Autodesk Fusion 360 part; units mm, degrees
(part 16 of 20)
  spline S45 degree 3 poles (25.501, -787.6508) (25.5046, -787.8666) (25.5109, -788.2453) (25.6995, -788.5712) (25.7807, -788.7115) knots 0 0 0 0 0.063398 0.111295 0.111295 0.111295 0.111295
  spline S46 degree 3 poles (25.7807, -788.7115) (25.8819, -788.808) (26.0864, -789.0031) (26.3682, -789.0291) (26.5106, -789.0423) knots 0 0 0 0 0.040675 0.082263 0.082263 0.082263 0.082263
  spline S47 degree 3 poles (26.5106, -789.0423) (26.625, -789.0341) (26.8478, -789.018) (27.0271, -788.8852) (27.1143, -788.8205) knots 0 0 0 0 0.033628 0.065508 0.065508 0.065508 0.065508
  spline S48 degree 3 poles (27.1143, -788.8205) (27.1883, -788.7306) (27.3518, -788.5319) (27.3967, -788.2775) (27.4212, -788.1384) knots 0 0 0 0 0.034396 0.07593 0.07593 0.07593 0.07593
  spline S49 degree 3 poles (21.7321, -737.034) (21.7357, -736.7657) (21.7422, -736.2825) (21.8615, -735.8147) (21.9145, -735.6066) knots 0 0 0 0 0.080152 0.144341 0.144341 0.144341 0.144341
  spline S50 degree 3 poles (21.9145, -735.6066) (21.9791, -735.4398) (22.1017, -735.1233) (22.3428, -734.8853) (22.4568, -734.7727) knots 0 0 0 0 0.052977 0.10048 0.10048 0.10048 0.10048
  spline S51 degree 3 poles (22.4568, -734.7727) (22.5882, -734.6872) (22.863, -734.5083) (23.1911, -734.4893) (23.3623, -734.4794) knots 0 0 0 0 0.046203 0.096661 0.096661 0.096661 0.096661
  spline S52 degree 3 poles (23.3623, -734.4794) (23.4901, -734.485) (23.7356, -734.4957) (23.9605, -734.5941) (24.0683, -734.6414) knots 0 0 0 0 0.037989 0.072993 0.072993 0.072993 0.072993
  spline S53 degree 3 poles (24.0683, -734.6414) (24.1655, -734.7021) (24.3629, -734.8252) (24.5001, -735.0132) (24.5697, -735.1086) knots 0 0 0 0 0.034048 0.069103 0.069103 0.069103 0.069103
  spline S54 degree 3 poles (24.5697, -735.1086) (24.633, -735.2196) (24.767, -735.4545) (24.841, -735.7148) (24.8801, -735.8521) knots 0 0 0 0 0.038176 0.080832 0.080832 0.080832 0.080832
  spline S55 degree 3 poles (24.8801, -735.8521) (24.9128, -736.0232) (24.9874, -736.4133) (24.9907, -736.8107) (24.9926, -737.0339) knots 0 0 0 0 0.052146 0.118926 0.118926 0.118926 0.118926
  spline S56 degree 3 poles (24.9926, -737.0339) (24.989, -737.3005) (24.9824, -737.7813) (24.8645, -738.247) (24.8119, -738.4544) knots 0 0 0 0 0.079639 0.143634 0.143634 0.143634 0.143634
  spline S57 degree 3 poles (24.8119, -738.4544) (24.7477, -738.6214) (24.6259, -738.9384) (24.3852, -739.1771) (24.2713, -739.2901) knots 0 0 0 0 0.052961 0.100531 0.100531 0.100531 0.100531
  spline S58 degree 3 poles (24.2713, -739.2901) (24.1397, -739.3761) (23.864, -739.5562) (23.5346, -739.5752) (23.3624, -739.5851) knots 0 0 0 0 0.046339 0.097057 0.097057 0.097057 0.097057
  spline S59 degree 3 poles (23.3624, -739.5851) (23.1362, -739.5658) (22.6949, -739.5281) (22.3801, -739.2179) (22.2267, -739.0667) knots 0 0 0 0 0.065835 0.128409 0.128409 0.128409 0.128409
  spline S60 degree 3 poles (22.2267, -739.0667) (22.0832, -738.7986) (21.7456, -738.1676) (21.737, -737.4479) (21.7321, -737.034) knots 0 0 0 0 0.090022 0.211899 0.211899 0.211899 0.211899
  line L356 (28.1509, -738.173) -> (28.7546, -738.2514)
  spline S61 degree 3 poles (28.7546, -738.2514) (28.7119, -738.4453) (28.6302, -738.8171) (28.3717, -739.0954) (28.2481, -739.2286) knots 0 0 0 0 0.058356 0.111856 0.111856 0.111856 0.111856
  spline S62 degree 3 poles (28.2481, -739.2286) (28.1021, -739.3315) (27.802, -739.543) (27.4353, -739.5685) (27.2471, -739.5816) knots 0 0 0 0 0.052559 0.107965 0.107965 0.107965 0.107965
  spline S63 degree 3 poles (27.2471, -739.5816) (27.0141, -739.5641) (26.5625, -739.5302) (26.2182, -739.2373) (26.0517, -739.0956) knots 0 0 0 0 0.068154 0.132052 0.132052 0.132052 0.132052
  spline S64 degree 3 poles (26.0517, -739.0956) (25.9201, -738.9049) (25.6323, -738.4875) (25.6112, -737.9787) (25.5997, -737.7024) knots 0 0 0 0 0.068157 0.149141 0.149141 0.149141 0.149141
  spline S65 degree 3 poles (25.5997, -737.7024) (25.6061, -737.5171) (25.6181, -737.1646) (25.7375, -736.8331) (25.7941, -736.6758) knots 0 0 0 0 0.055211 0.105055 0.105055 0.105055 0.105055
  spline S66 degree 3 poles (25.7941, -736.6758) (25.8663, -736.5389) (26.0085, -736.2693) (26.2614, -736.0994) (26.3859, -736.0158) knots 0 0 0 0 0.04564 0.089884 0.089884 0.089884 0.089884
  spline S67 degree 3 poles (26.3859, -736.0158) (26.5218, -735.9516) (26.7957, -735.8223) (27.0981, -735.8047) (27.2505, -735.7958) knots 0 0 0 0 0.044643 0.089956 0.089956 0.089956 0.089956
  spline S68 degree 3 poles (27.2505, -735.7958) (27.4342, -735.8052) (27.7821, -735.8229) (28.0767, -736.0072) (28.2157, -736.0942) knots 0 0 0 0 0.054149 0.102527 0.102527 0.102527 0.102527
  spline S69 degree 3 poles (28.2157, -736.0942) (28.3301, -736.2077) (28.5692, -736.4447) (28.6529, -736.7715) (28.6966, -736.9417) knots 0 0 0 0 0.047449 0.099081 0.099081 0.099081 0.099081
  line L357 (28.6966, -736.9417) -> (28.0997, -737.0338)
  spline S70 degree 3 poles (28.0997, -737.0338) (28.0689, -736.9224) (28.0114, -736.715) (27.8654, -736.5576) (27.7979, -736.4847) knots 0 0 0 0 0.034086 0.063475 0.063475 0.063475 0.063475
  spline S71 degree 3 poles (27.7979, -736.4847) (27.7209, -736.431) (27.5636, -736.3213) (27.3721, -736.3076) (27.2743, -736.3006) knots 0 0 0 0 0.027619 0.056426 0.056426 0.056426 0.056426
  spline S72 degree 3 poles (27.2743, -736.3006) (27.1277, -736.3136) (26.8385, -736.3393) (26.6256, -736.5361) (26.5206, -736.6331) knots 0 0 0 0 0.04285 0.084486 0.084486 0.084486 0.084486
  spline S73 degree 3 poles (26.5206, -736.6331) (26.4364, -736.7727) (26.2425, -737.0942) (26.235, -737.4717) (26.2307, -737.6853) knots 0 0 0 0 0.048123 0.11083 0.11083 0.11083 0.11083
  spline S74 degree 3 poles (26.2307, -737.6853) (26.2343, -737.9011) (26.2406, -738.2798) (26.4292, -738.6057) (26.5104, -738.746) knots 0 0 0 0 0.063398 0.111295 0.111295 0.111295 0.111295
  spline S75 degree 3 poles (26.5104, -738.746) (26.6116, -738.8425) (26.8161, -739.0376) (27.0979, -739.0637) (27.2403, -739.0768) knots 0 0 0 0 0.040675 0.082263 0.082263 0.082263 0.082263
  spline S76 degree 3 poles (27.2403, -739.0768) (27.3547, -739.0686) (27.5775, -739.0526) (27.7568, -738.9198) (27.844, -738.8551) knots 0 0 0 0 0.033628 0.065508 0.065508 0.065508 0.065508
  spline S77 degree 3 poles (27.844, -738.8551) (27.918, -738.7651) (28.0815, -738.5665) (28.1264, -738.3121) (28.1509, -738.173) knots 0 0 0 0 0.034396 0.07593 0.07593 0.07593 0.07593
  line L358 (21.7306, -688.1902) -> (22.3752, -688.1357)
  spline S78 degree 3 poles (22.3752, -688.1357) (22.4029, -688.2789) (22.4541, -688.5438) (22.6279, -688.7491) (22.7077, -688.8434) knots 0 0 0 0 0.042908 0.079365 0.079365 0.079365 0.079365
  spline S79 degree 3 poles (22.7077, -688.8434) (22.7999, -688.9125) (22.9865, -689.0525) (23.2192, -689.071) (23.337, -689.0804) knots 0 0 0 0 0.033826 0.068485 0.068485 0.068485 0.068485
  spline S80 degree 3 poles (23.337, -689.0804) (23.4794, -689.0661) (23.7662, -689.0373) (23.9798, -688.8436) (24.0873, -688.7462) knots 0 0 0 0 0.041772 0.0841 0.0841 0.0841 0.0841
  spline S81 degree 3 poles (24.0873, -688.7462) (24.1768, -688.6211) (24.366, -688.3566) (24.3845, -688.031) (24.3943, -687.8594) knots 0 0 0 0 0.045186 0.095569 0.095569 0.095569 0.095569
  spline S82 degree 3 poles (24.3943, -687.8594) (24.3852, -687.697) (24.3681, -687.3907) (24.1852, -687.1457) (24.0992, -687.0306) knots 0 0 0 0 0.047557 0.089725 0.089725 0.089725 0.089725
  spline S83 degree 3 poles (24.0992, -687.0306) (23.9907, -686.9421) (23.7662, -686.7589) (23.4765, -686.7379) (23.3267, -686.7271) knots 0 0 0 0 0.040971 0.08482 0.08482 0.08482 0.08482
  spline S84 degree 3 poles (23.3267, -686.7271) (23.2311, -686.7322) (23.0437, -686.7423) (22.8742, -686.8225) (22.7912, -686.8618) knots 0 0 0 0 0.028423 0.055689 0.055689 0.055689 0.055689
  spline S85 degree 3 poles (22.7912, -686.8618) (22.7164, -686.9093) (22.5695, -687.0026) (22.4666, -687.1427) (22.4161, -687.2114) knots 0 0 0 0 0.026342 0.051681 0.051681 0.051681 0.051681
  line L359 (22.4161, -687.2114) -> (21.8397, -687.1364)
  line L360 (21.8397, -687.1364) -> (22.324, -684.5681)
  line L361 (22.324, -684.5681) -> (24.8103, -684.5681)
  line L362 (24.8103, -684.5681) -> (24.8103, -685.1547)
  line L363 (24.8103, -685.1547) -> (22.8151, -685.1548)
  line L364 (22.8151, -685.1548) -> (22.5457, -686.4986)
  spline S86 degree 3 poles (22.5457, -686.4986) (22.6952, -686.4071) (22.986, -686.229) (23.3254, -686.1992) (23.4904, -686.1848) knots 0 0 0 0 0.051785 0.100763 0.100763 0.100763 0.100763
  spline S87 degree 3 poles (23.4904, -686.1848) (23.6997, -686.2031) (24.1153, -686.2396) (24.4361, -686.5061) (24.5955, -686.6384) knots 0 0 0 0 0.061424 0.122014 0.122014 0.122014 0.122014
  spline S88 degree 3 poles (24.5955, -686.6384) (24.7267, -686.8038) (24.9976, -687.1451) (25.0293, -687.5805) (25.0457, -687.8048) knots 0 0 0 0 0.061868 0.127641 0.127641 0.127641 0.127641
  spline S89 degree 3 poles (25.0457, -687.8048) (25.0305, -688.0218) (25.0006, -688.4476) (24.7654, -688.8035) (24.6501, -688.9781) knots 0 0 0 0 0.064036 0.125703 0.125703 0.125703 0.125703
  spline S90 degree 3 poles (24.6501, -688.9781) (24.4723, -689.1551) (24.1093, -689.5168) (23.598, -689.5621) (23.337, -689.5852) knots 0 0 0 0 0.072854 0.148822 0.148822 0.148822 0.148822
  spline S91 degree 3 poles (23.337, -689.5852) (23.1238, -689.5724) (22.7162, -689.5481) (22.3825, -689.3145) (22.2234, -689.2032) knots 0 0 0 0 0.062678 0.119794 0.119794 0.119794 0.119794
  spline S92 degree 3 poles (22.2234, -689.2032) (22.0948, -689.0628) (21.8305, -688.7745) (21.7644, -688.3884) (21.7306, -688.1902) knots 0 0 0 0 0.055877 0.114795 0.114795 0.114795 0.114795
  line L365 (28.1494, -688.1731) -> (28.7531, -688.2516)
  spline S93 degree 3 poles (28.7531, -688.2516) (28.7104, -688.4455) (28.6286, -688.8172) (28.3702, -689.0956) (28.2466, -689.2287) knots 0 0 0 0 0.058356 0.111856 0.111856 0.111856 0.111856
  spline S94 degree 3 poles (28.2466, -689.2287) (28.1005, -689.3317) (27.8004, -689.5431) (27.4337, -689.5686) (27.2456, -689.5817) knots 0 0 0 0 0.052559 0.107965 0.107965 0.107965 0.107965
  spline S95 degree 3 poles (27.2456, -689.5817) (27.0125, -689.5642) (26.5609, -689.5303) (26.2167, -689.2374) (26.0501, -689.0957) knots 0 0 0 0 0.068154 0.132052 0.132052 0.132052 0.132052
  spline S96 degree 3 poles (26.0501, -689.0957) (25.9186, -688.905) (25.6307, -688.4876) (25.6097, -687.9788) (25.5982, -687.7025) knots 0 0 0 0 0.068157 0.149141 0.149141 0.149141 0.149141
  spline S97 degree 3 poles (25.5982, -687.7025) (25.6045, -687.5172) (25.6165, -687.1647) (25.7359, -686.8332) (25.7926, -686.6759) knots 0 0 0 0 0.055211 0.105055 0.105055 0.105055 0.105055
  spline S98 degree 3 poles (25.7926, -686.6759) (25.8648, -686.539) (26.007, -686.2694) (26.2599, -686.0995) (26.3843, -686.0159) knots 0 0 0 0 0.04564 0.089884 0.089884 0.089884 0.089884
  spline S99 degree 3 poles (26.3843, -686.0159) (26.5203, -685.9517) (26.7942, -685.8225) (27.0966, -685.8048) (27.2489, -685.7959) knots 0 0 0 0 0.044643 0.089955 0.089955 0.089955 0.089955
  spline S100 degree 3 poles (27.2489, -685.7959) (27.4327, -685.8053) (27.7805, -685.8231) (28.0751, -686.0074) (28.2142, -686.0943) knots 0 0 0 0 0.054149 0.102527 0.102527 0.102527 0.102527
  spline S101 degree 3 poles (28.2142, -686.0943) (28.3286, -686.2078) (28.5677, -686.4449) (28.6514, -686.7716) (28.6951, -686.9419) knots 0 0 0 0 0.047449 0.099081 0.099081 0.099081 0.099081
  line L366 (28.6951, -686.9419) -> (28.0982, -687.034)
  spline S102 degree 3 poles (28.0982, -687.034) (28.0673, -686.9226) (28.0099, -686.7151) (27.8639, -686.5577) (27.7964, -686.4849) knots 0 0 0 0 0.034086 0.063475 0.063475 0.063475 0.063475
  spline S103 degree 3 poles (27.7964, -686.4849) (27.7194, -686.4311) (27.5621, -686.3214) (27.3706, -686.3077) (27.2728, -686.3007) knots 0 0 0 0 0.027619 0.056426 0.056426 0.056426 0.056426
  spline S104 degree 3 poles (27.2728, -686.3007) (27.1262, -686.3137) (26.837, -686.3394) (26.624, -686.5362) (26.5191, -686.6332) knots 0 0 0 0 0.04285 0.084486 0.084486 0.084486 0.084486
  spline S105 degree 3 poles (26.5191, -686.6332) (26.4349, -686.7728) (26.241, -687.0943) (26.2335, -687.4718) (26.2292, -687.6854) knots 0 0 0 0 0.048123 0.11083 0.11083 0.11083 0.11083
  spline S106 degree 3 poles (26.2292, -687.6854) (26.2328, -687.9012) (26.2391, -688.2799) (26.4277, -688.6059) (26.5089, -688.7461) knots 0 0 0 0 0.063398 0.111295 0.111295 0.111295 0.111295
  spline S107 degree 3 poles (26.5089, -688.7461) (26.61, -688.8426) (26.8146, -689.0378) (27.0963, -689.0638) (27.2387, -689.0769) knots 0 0 0 0 0.040675 0.082263 0.082263 0.082263 0.082263
  spline S108 degree 3 poles (27.2387, -689.0769) (27.3531, -689.0687) (27.576, -689.0527) (27.7552, -688.9199) (27.8424, -688.8553) knots 0 0 0 0 0.033628 0.065508 0.065508 0.065508 0.065508
  spline S109 degree 3 poles (27.8424, -688.8553) (27.9165, -688.7653) (28.0799, -688.5666) (28.1248, -688.3123) (28.1494, -688.1731) knots 0 0 0 0 0.034396 0.07593 0.07593 0.07593 0.07593
  spline S110 degree 3 poles (22.0101, -637.034) (22.0137, -636.7656) (22.0202, -636.2824) (22.1394, -635.8146) (22.1925, -635.6066) knots 0 0 0 0 0.080152 0.144341 0.144341 0.144341 0.144341
  spline S111 degree 3 poles (22.1925, -635.6066) (22.2571, -635.4397) (22.3796, -635.1233) (22.6208, -634.8852) (22.7348, -634.7727) knots 0 0 0 0 0.052977 0.10048 0.10048 0.10048 0.10048
  spline S112 degree 3 poles (22.7348, -634.7727) (22.8661, -634.6872) (23.141, -634.5083) (23.469, -634.4893) (23.6403, -634.4794) knots 0 0 0 0 0.046203 0.096661 0.096661 0.096661 0.096661
  spline S113 degree 3 poles (23.6403, -634.4794) (23.7681, -634.4849) (24.0136, -634.4956) (24.2384, -634.5941) (24.3463, -634.6413) knots 0 0 0 0 0.037989 0.072993 0.072993 0.072993 0.072993
  spline S114 degree 3 poles (24.3463, -634.6413) (24.4435, -634.702) (24.6409, -634.8252) (24.7781, -635.0132) (24.8477, -635.1086) knots 0 0 0 0 0.034048 0.069103 0.069103 0.069103 0.069103
  spline S115 degree 3 poles (24.8477, -635.1086) (24.911, -635.2195) (25.045, -635.4544) (25.119, -635.7147) (25.1581, -635.8521) knots 0 0 0 0 0.038176 0.080832 0.080832 0.080832 0.080832
  spline S116 degree 3 poles (25.1581, -635.8521) (25.1908, -636.0231) (25.2653, -636.4133) (25.2687, -636.8107) (25.2706, -637.0339) knots 0 0 0 0 0.052146 0.118926 0.118926 0.118926 0.118926
  spline S117 degree 3 poles (25.2706, -637.0339) (25.267, -637.3005) (25.2604, -637.7813) (25.1425, -638.2469) (25.0899, -638.4544) knots 0 0 0 0 0.079639 0.143634 0.143634 0.143634 0.143634
  spline S118 degree 3 poles (25.0899, -638.4544) (25.0257, -638.6214) (24.9039, -638.9383) (24.6632, -639.1771) (24.5493, -639.29) knots 0 0 0 0 0.052961 0.100531 0.100531 0.100531 0.100531
  spline S119 degree 3 poles (24.5493, -639.29) (24.4177, -639.376) (24.142, -639.5562) (23.8126, -639.5752) (23.6404, -639.5851) knots 0 0 0 0 0.046339 0.097057 0.097057 0.097057 0.097057
  spline S120 degree 3 poles (23.6404, -639.5851) (23.4142, -639.5658) (22.9729, -639.5281) (22.6581, -639.2179) (22.5047, -639.0667) knots 0 0 0 0 0.065835 0.128409 0.128409 0.128409 0.128409
  spline S121 degree 3 poles (22.5047, -639.0667) (22.3612, -638.7986) (22.0236, -638.1676) (22.015, -637.4479) (22.0101, -637.034) knots 0 0 0 0 0.090022 0.211899 0.211899 0.211899 0.211899
  line L367 (28.4289, -638.1729) -> (29.0326, -638.2514)
  spline S122 degree 3 poles (29.0326, -638.2514) (28.9899, -638.4453) (28.9082, -638.817) (28.6498, -639.0954) (28.5262, -639.2285) knots 0 0 0 0 0.058356 0.111856 0.111856 0.111856 0.111856
  spline S123 degree 3 poles (28.5262, -639.2285) (28.3801, -639.3315) (28.08, -639.5429) (27.7133, -639.5685) (27.5251, -639.5816) knots 0 0 0 0 0.052559 0.107965 0.107965 0.107965 0.107965
  spline S124 degree 3 poles (27.5251, -639.5816) (27.2921, -639.5641) (26.8405, -639.5301) (26.4963, -639.2373) (26.3297, -639.0956) knots 0 0 0 0 0.068154 0.132052 0.132052 0.132052 0.132052
  spline S125 degree 3 poles (26.3297, -639.0956) (26.1981, -638.9048) (25.9103, -638.4875) (25.8892, -637.9786) (25.8777, -637.7023) knots 0 0 0 0 0.068157 0.149141 0.149141 0.149141 0.149141
  spline S126 degree 3 poles (25.8777, -637.7023) (25.8841, -637.5171) (25.8961, -637.1646) (26.0155, -636.833) (26.0721, -636.6757) knots 0 0 0 0 0.055211 0.105055 0.105055 0.105055 0.105055
  spline S127 degree 3 poles (26.0721, -636.6757) (26.1443, -636.5388) (26.2865, -636.2692) (26.5394, -636.0994) (26.6639, -636.0158) knots 0 0 0 0 0.04564 0.089884 0.089884 0.089884 0.089884
  spline S128 degree 3 poles (26.6639, -636.0158) (26.7998, -635.9516) (27.0737, -635.8223) (27.3761, -635.8046) (27.5284, -635.7958) knots 0 0 0 0 0.044643 0.089955 0.089955 0.089955 0.089955
  spline S129 degree 3 poles (27.5284, -635.7958) (27.7122, -635.8051) (28.0601, -635.8229) (28.3547, -636.0072) (28.4937, -636.0942) knots 0 0 0 0 0.054149 0.102527 0.102527 0.102527 0.102527
  spline S130 degree 3 poles (28.4937, -636.0942) (28.6081, -636.2077) (28.8472, -636.4447) (28.9309, -636.7714) (28.9746, -636.9417) knots 0 0 0 0 0.047449 0.099081 0.099081 0.099081 0.099081
  line L368 (28.9746, -636.9417) -> (28.3777, -637.0338)
  spline S131 degree 3 poles (28.3777, -637.0338) (28.3469, -636.9224) (28.2894, -636.715) (28.1434, -636.5576) (28.0759, -636.4847) knots 0 0 0 0 0.034086 0.063475 0.063475 0.063475 0.063475
  spline S132 degree 3 poles (28.0759, -636.4847) (27.9989, -636.431) (27.8416, -636.3213) (27.6501, -636.3075) (27.5523, -636.3005) knots 0 0 0 0 0.027619 0.056426 0.056426 0.056426 0.056426
  spline S133 degree 3 poles (27.5523, -636.3005) (27.4057, -636.3136) (27.1165, -636.3393) (26.9036, -636.5361) (26.7986, -636.6331) knots 0 0 0 0 0.04285 0.084486 0.084486 0.084486 0.084486
  spline S134 degree 3 poles (26.7986, -636.6331) (26.7144, -636.7727) (26.5205, -637.0941) (26.513, -637.4717) (26.5087, -637.6853) knots 0 0 0 0 0.048123 0.11083 0.11083 0.11083 0.11083
  spline S135 degree 3 poles (26.5087, -637.6853) (26.5123, -637.901) (26.5186, -638.2798) (26.7072, -638.6057) (26.7884, -638.746) knots 0 0 0 0 0.063398 0.111295 0.111295 0.111295 0.111295
  spline S136 degree 3 poles (26.7884, -638.746) (26.8896, -638.8425) (27.0941, -639.0376) (27.3759, -639.0636) (27.5183, -639.0768) knots 0 0 0 0 0.040675 0.082263 0.082263 0.082263 0.082263
  spline S137 degree 3 poles (27.5183, -639.0768) (27.6327, -639.0686) (27.8555, -639.0526) (28.0348, -638.9197) (28.122, -638.8551) knots 0 0 0 0 0.033628 0.065508 0.065508 0.065508 0.065508
  spline S138 degree 3 poles (28.122, -638.8551) (28.196, -638.7651) (28.3595, -638.5665) (28.4044, -638.3121) (28.4289, -638.1729) knots 0 0 0 0 0.034396 0.07593 0.07593 0.07593 0.07593
  line L369 (22.0076, -588.1903) -> (22.6523, -588.1357)
  spline S139 degree 3 poles (22.6523, -588.1357) (22.68, -588.2789) (22.7312, -588.5439) (22.905, -588.7491) (22.9848, -588.8434) knots 0 0 0 0 0.042908 0.079365 0.079365 0.079365 0.079365
  spline S140 degree 3 poles (22.9848, -588.8434) (23.077, -588.9125) (23.2636, -589.0525) (23.4963, -589.0711) (23.6141, -589.0804) knots 0 0 0 0 0.033826 0.068485 0.068485 0.068485 0.068485
  spline S141 degree 3 poles (23.6141, -589.0804) (23.7565, -589.0662) (24.0433, -589.0374) (24.2569, -588.8437) (24.3644, -588.7462) knots 0 0 0 0 0.041772 0.0841 0.0841 0.0841 0.0841
  spline S142 degree 3 poles (24.3644, -588.7462) (24.4539, -588.6211) (24.6431, -588.3567) (24.6616, -588.0311) (24.6714, -587.8594) knots 0 0 0 0 0.045186 0.095569 0.095569 0.095569 0.095569
  spline S143 degree 3 poles (24.6714, -587.8594) (24.6623, -587.6971) (24.6452, -587.3908) (24.4623, -587.1458) (24.3763, -587.0306) knots 0 0 0 0 0.047557 0.089725 0.089725 0.089725 0.089725
  spline S144 degree 3 poles (24.3763, -587.0306) (24.2678, -586.9421) (24.0433, -586.7589) (23.7536, -586.7379) (23.6038, -586.7271) knots 0 0 0 0 0.040971 0.08482 0.08482 0.08482 0.08482
  spline S145 degree 3 poles (23.6038, -586.7271) (23.5082, -586.7322) (23.3208, -586.7423) (23.1513, -586.8225) (23.0683, -586.8618) knots 0 0 0 0 0.028423 0.055689 0.055689 0.055689 0.055689
  spline S146 degree 3 poles (23.0683, -586.8618) (22.9935, -586.9094) (22.8466, -587.0026) (22.7437, -587.1427) (22.6932, -587.2114) knots 0 0 0 0 0.026342 0.051681 0.051681 0.051681 0.051681
  line L370 (22.6932, -587.2114) -> (22.1168, -587.1364)
  line L371 (22.1168, -587.1364) -> (22.6011, -584.5682)
  line L372 (22.6011, -584.5682) -> (25.0874, -584.5682)
  line L373 (25.0874, -584.5682) -> (25.0874, -585.1548)
  line L374 (25.0874, -585.1548) -> (23.0922, -585.1548)
  line L375 (23.0922, -585.1548) -> (22.8228, -586.4986)
  spline S147 degree 3 poles (22.8228, -586.4986) (22.9723, -586.4071) (23.2631, -586.2291) (23.6026, -586.1993) (23.7675, -586.1848) knots 0 0 0 0 0.051785 0.100763 0.100763 0.100763 0.100763
  spline S148 degree 3 poles (23.7675, -586.1848) (23.9768, -586.2032) (24.3924, -586.2397) (24.7132, -586.5061) (24.8726, -586.6384) knots 0 0 0 0 0.061424 0.122014 0.122014 0.122014 0.122014
  spline S149 degree 3 poles (24.8726, -586.6384) (25.0039, -586.8039) (25.2747, -587.1452) (25.3064, -587.5805) (25.3228, -587.8049) knots 0 0 0 0 0.061868 0.12764 0.12764 0.12764 0.12764
  spline S150 degree 3 poles (25.3228, -587.8049) (25.3076, -588.0218) (25.2777, -588.4477) (25.0425, -588.8035) (24.9272, -588.9781) knots 0 0 0 0 0.064036 0.125703 0.125703 0.125703 0.125703
  spline S151 degree 3 poles (24.9272, -588.9781) (24.7494, -589.1552) (24.3864, -589.5168) (23.8751, -589.5621) (23.6141, -589.5852) knots 0 0 0 0 0.072854 0.148822 0.148822 0.148822 0.148822
  spline S152 degree 3 poles (23.6141, -589.5852) (23.4008, -589.5725) (22.9933, -589.5481) (22.6596, -589.3146) (22.5005, -589.2032) knots 0 0 0 0 0.062678 0.119794 0.119794 0.119794 0.119794
  spline S153 degree 3 poles (22.5005, -589.2032) (22.3719, -589.0629) (22.1076, -588.7745) (22.0415, -588.3884) (22.0076, -588.1903) knots 0 0 0 0 0.055877 0.114795 0.114795 0.114795 0.114795
  line L376 (28.4265, -588.1732) -> (29.0302, -588.2516)
  spline S154 degree 3 poles (29.0302, -588.2516) (28.9875, -588.4456) (28.9057, -588.8173) (28.6473, -589.0956) (28.5237, -589.2288) knots 0 0 0 0 0.058356 0.111856 0.111856 0.111856 0.111856
  spline S155 degree 3 poles (28.5237, -589.2288) (28.3776, -589.3317) (28.0775, -589.5432) (27.7108, -589.5687) (27.5227, -589.5818) knots 0 0 0 0 0.052559 0.107965 0.107965 0.107965 0.107965
  spline S156 degree 3 poles (27.5227, -589.5818) (27.2896, -589.5643) (26.838, -589.5304) (26.4938, -589.2375) (26.3272, -589.0958) knots 0 0 0 0 0.068154 0.132052 0.132052 0.132052 0.132052
  spline S157 degree 3 poles (26.3272, -589.0958) (26.1957, -588.905) (25.9078, -588.4877) (25.8867, -587.9788) (25.8753, -587.7025) knots 0 0 0 0 0.068157 0.149141 0.149141 0.149141 0.149141
  spline S158 degree 3 poles (25.8753, -587.7025) (25.8816, -587.5173) (25.8936, -587.1648) (26.013, -586.8332) (26.0697, -586.6759) knots 0 0 0 0 0.055211 0.105055 0.105055 0.105055 0.105055
  spline S159 degree 3 poles (26.0697, -586.6759) (26.1419, -586.539) (26.2841, -586.2694) (26.537, -586.0996) (26.6615, -586.016) knots 0 0 0 0 0.04564 0.089884 0.089884 0.089884 0.089884
  spline S160 degree 3 poles (26.6615, -586.016) (26.7974, -585.9518) (27.0713, -585.8225) (27.3737, -585.8049) (27.526, -585.796) knots 0 0 0 0 0.044643 0.089955 0.089955 0.089955 0.089955
  spline S161 degree 3 poles (27.526, -585.796) (27.7098, -585.8054) (28.0577, -585.8231) (28.3523, -586.0074) (28.4913, -586.0944) knots 0 0 0 0 0.054149 0.102527 0.102527 0.102527 0.102527
  spline S162 degree 3 poles (28.4913, -586.0944) (28.6057, -586.2079) (28.8448, -586.4449) (28.9285, -586.7717) (28.9722, -586.9419) knots 0 0 0 0 0.047449 0.099081 0.099081 0.099081 0.099081
  line L377 (28.9722, -586.9419) -> (28.3753, -587.034)
  spline S163 degree 3 poles (28.3753, -587.034) (28.3444, -586.9226) (28.287, -586.7152) (28.141, -586.5578) (28.0735, -586.4849) knots 0 0 0 0 0.034086 0.063475 0.063475 0.063475 0.063475
  spline S164 degree 3 poles (28.0735, -586.4849) (27.9965, -586.4312) (27.8392, -586.3215) (27.6477, -586.3078) (27.5499, -586.3008) knots 0 0 0 0 0.027619 0.056426 0.056426 0.056426 0.056426
  spline S165 degree 3 poles (27.5499, -586.3008) (27.4033, -586.3138) (27.1141, -586.3395) (26.9011, -586.5363) (26.7962, -586.6333) knots 0 0 0 0 0.04285 0.084486 0.084486 0.084486 0.084486
  spline S166 degree 3 poles (26.7962, -586.6333) (26.712, -586.7729) (26.5181, -587.0943) (26.5106, -587.4719) (26.5063, -587.6855) knots 0 0 0 0 0.048123 0.11083 0.11083 0.11083 0.11083
  spline S167 degree 3 poles (26.5063, -587.6855) (26.5099, -587.9012) (26.5162, -588.28) (26.7048, -588.6059) (26.786, -588.7462) knots 0 0 0 0 0.063398 0.111295 0.111295 0.111295 0.111295
  spline S168 degree 3 poles (26.786, -588.7462) (26.8871, -588.8427) (27.0917, -589.0378) (27.3734, -589.0639) (27.5158, -589.077) knots 0 0 0 0 0.040675 0.082263 0.082263 0.082263 0.082263
  spline S169 degree 3 poles (27.5158, -589.077) (27.6302, -589.0688) (27.8531, -589.0528) (28.0323, -588.92) (28.1195, -588.8553) knots 0 0 0 0 0.033628 0.065508 0.065508 0.065508 0.065508
  spline S170 degree 3 poles (28.1195, -588.8553) (28.1936, -588.7653) (28.357, -588.5667) (28.4019, -588.3123) (28.4265, -588.1732) knots 0 0 0 0 0.034396 0.07593 0.07593 0.07593 0.07593
  spline S171 degree 3 poles (21.9704, -537.0337) (21.974, -536.7654) (21.9805, -536.2822) (22.0997, -535.8144) (22.1528, -535.6063) knots 0 0 0 0 0.080152 0.144341 0.144341 0.144341 0.144341
  spline S172 degree 3 poles (22.1528, -535.6063) (22.2174, -535.4395) (22.3399, -535.123) (22.581, -534.8849) (22.695, -534.7724) knots 0 0 0 0 0.052977 0.10048 0.10048 0.10048 0.10048
  spline S173 degree 3 poles (22.695, -534.7724) (22.8264, -534.6869) (23.1012, -534.508) (23.4293, -534.4889) (23.6005, -534.479) knots 0 0 0 0 0.046203 0.096661 0.096661 0.096661 0.096661
  spline S174 degree 3 poles (23.6005, -534.479) (23.7283, -534.4846) (23.9738, -534.4953) (24.1987, -534.5937) (24.3065, -534.6409) knots 0 0 0 0 0.037989 0.072993 0.072993 0.072993 0.072993
  spline S175 degree 3 poles (24.3065, -534.6409) (24.4038, -534.7016) (24.6011, -534.8248) (24.7383, -535.0128) (24.8079, -535.1082) knots 0 0 0 0 0.034048 0.069103 0.069103 0.069103 0.069103
  spline S176 degree 3 poles (24.8079, -535.1082) (24.8712, -535.2191) (25.0053, -535.454) (25.0793, -535.7143) (25.1184, -535.8517) knots 0 0 0 0 0.038176 0.080832 0.080832 0.080832 0.080832
  spline S177 degree 3 poles (25.1184, -535.8517) (25.1511, -536.0227) (25.2257, -536.4128) (25.2291, -536.8103) (25.231, -537.0334) knots 0 0 0 0 0.052146 0.118926 0.118926 0.118926 0.118926
  spline S178 degree 3 poles (25.231, -537.0334) (25.2274, -537.3) (25.2208, -537.7808) (25.1029, -538.2465) (25.0504, -538.454) knots 0 0 0 0 0.079639 0.143634 0.143634 0.143634 0.143634
  spline S179 degree 3 poles (25.0504, -538.454) (24.9862, -538.6209) (24.8644, -538.9379) (24.6237, -539.1767) (24.5098, -539.2896) knots 0 0 0 0 0.052961 0.100531 0.100531 0.100531 0.100531
  spline S180 degree 3 poles (24.5098, -539.2896) (24.3782, -539.3756) (24.1025, -539.5558) (23.7731, -539.5748) (23.6009, -539.5847) knots 0 0 0 0 0.046339 0.097057 0.097057 0.097057 0.097057
  spline S181 degree 3 poles (23.6009, -539.5847) (23.3747, -539.5654) (22.9334, -539.5278) (22.6186, -539.2176) (22.4651, -539.0664) knots 0 0 0 0 0.065835 0.128409 0.128409 0.128409 0.128409
  spline S182 degree 3 poles (22.4651, -539.0664) (22.3217, -538.7983) (21.984, -538.1673) (21.9754, -537.4476) (21.9704, -537.0337) knots 0 0 0 0 0.090022 0.211899 0.211899 0.211899 0.211899
  line L378 (28.3894, -538.1723) -> (28.993, -538.2507)
  spline S183 degree 3 poles (28.993, -538.2507) (28.9504, -538.4446) (28.8686, -538.8163) (28.6102, -539.0947) (28.4866, -539.2279) knots 0 0 0 0 0.058356 0.111856 0.111856 0.111856 0.111856
  spline S184 degree 3 poles (28.4866, -539.2279) (28.3406, -539.3309) (28.0405, -539.5423) (27.6738, -539.5679) (27.4857, -539.581) knots 0 0 0 0 0.052559 0.107965 0.107965 0.107965 0.107965
  spline S185 degree 3 poles (27.4857, -539.581) (27.2526, -539.5635) (26.801, -539.5296) (26.4568, -539.2368) (26.2902, -539.0951) knots 0 0 0 0 0.068154 0.132052 0.132052 0.132052 0.132052
  spline S186 degree 3 poles (26.2902, -539.0951) (26.1586, -538.9043) (25.8707, -538.487) (25.8496, -537.9782) (25.8382, -537.7019) knots 0 0 0 0 0.068157 0.149141 0.149141 0.149141 0.149141
  spline S187 degree 3 poles (25.8382, -537.7019) (25.8445, -537.5166) (25.8564, -537.1641) (25.9758, -536.8326) (26.0325, -536.6752) knots 0 0 0 0 0.055211 0.105055 0.105055 0.105055 0.105055
  spline S188 degree 3 poles (26.0325, -536.6752) (26.1047, -536.5383) (26.2468, -536.2687) (26.4997, -536.0988) (26.6242, -536.0152) knots 0 0 0 0 0.04564 0.089884 0.089884 0.089884 0.089884
  spline S189 degree 3 poles (26.6242, -536.0152) (26.7601, -535.9511) (27.034, -535.8218) (27.3364, -535.8041) (27.4887, -535.7952) knots 0 0 0 0 0.044643 0.089956 0.089956 0.089956 0.089956
  spline S190 degree 3 poles (27.4887, -535.7952) (27.6725, -535.8045) (28.0203, -535.8223) (28.315, -536.0066) (28.454, -536.0935) knots 0 0 0 0 0.054149 0.102527 0.102527 0.102527 0.102527
  spline S191 degree 3 poles (28.454, -536.0935) (28.5685, -536.207) (28.8075, -536.444) (28.8913, -536.7708) (28.935, -536.941) knots 0 0 0 0 0.047449 0.099081 0.099081 0.099081 0.099081
  line L379 (28.935, -536.941) -> (28.3381, -537.0332)
  spline S192 degree 3 poles (28.3381, -537.0332) (28.3072, -536.9218) (28.2497, -536.7143) (28.1038, -536.557) (28.0362, -536.4841) knots 0 0 0 0 0.034086 0.063475 0.063475 0.063475 0.063475
  spline S193 degree 3 poles (28.0362, -536.4841) (27.9592, -536.4304) (27.8019, -536.3207) (27.6104, -536.3069) (27.5127, -536.2999) knots 0 0 0 0 0.027619 0.056426 0.056426 0.056426 0.056426
  spline S194 degree 3 poles (27.5127, -536.2999) (27.366, -536.313) (27.0769, -536.3387) (26.8639, -536.5356) (26.7589, -536.6325) knots 0 0 0 0 0.04285 0.084486 0.084486 0.084486 0.084486
  spline S195 degree 3 poles (26.7589, -536.6325) (26.6748, -536.7721) (26.4809, -537.0936) (26.4734, -537.4712) (26.4691, -537.6848) knots 0 0 0 0 0.048123 0.11083 0.11083 0.11083 0.11083
  spline S196 degree 3 poles (26.4691, -537.6848) (26.4727, -537.9005) (26.4791, -538.2793) (26.6677, -538.6052) (26.7489, -538.7454) knots 0 0 0 0 0.063398 0.111295 0.111295 0.111295 0.111295
  spline S197 degree 3 poles (26.7489, -538.7454) (26.85, -538.8419) (27.0546, -539.037) (27.3364, -539.0631) (27.4788, -539.0762) knots 0 0 0 0 0.040675 0.082263 0.082263 0.082263 0.082263
  spline S198 degree 3 poles (27.4788, -539.0762) (27.5932, -539.068) (27.816, -539.052) (27.9952, -538.9191) (28.0825, -538.8545) knots 0 0 0 0 0.033628 0.065508 0.065508 0.065508 0.065508
  spline S199 degree 3 poles (28.0825, -538.8545) (28.1565, -538.7645) (28.32, -538.5658) (28.3648, -538.3115) (28.3894, -538.1723) knots 0 0 0 0 0.034396 0.07593 0.07593 0.07593 0.07593
  line L380 (21.9641, -488.1903) -> (22.6087, -488.1357)
  spline S200 degree 3 poles (22.6087, -488.1357) (22.6364, -488.2789) (22.6877, -488.5438) (22.8614, -488.7491) (22.9413, -488.8434) knots 0 0 0 0 0.042908 0.079365 0.079365 0.079365 0.079365
  spline S201 degree 3 poles (22.9413, -488.8434) (23.0334, -488.9125) (23.2201, -489.0525) (23.4528, -489.071) (23.5705, -489.0804) knots 0 0 0 0 0.033826 0.068485 0.068485 0.068485 0.068485
  spline S202 degree 3 poles (23.5705, -489.0804) (23.713, -489.0661) (23.9997, -489.0373) (24.2134, -488.8436) (24.3209, -488.7461) knots 0 0 0 0 0.041772 0.0841 0.0841 0.0841 0.0841
  spline S203 degree 3 poles (24.3209, -488.7461) (24.4103, -488.6211) (24.5995, -488.3566) (24.618, -488.031) (24.6278, -487.8594) knots 0 0 0 0 0.045186 0.095569 0.095569 0.095569 0.095569
  spline S204 degree 3 poles (24.6278, -487.8594) (24.6187, -487.697) (24.6017, -487.3907) (24.4187, -487.1457) (24.3328, -487.0306) knots 0 0 0 0 0.047557 0.089725 0.089725 0.089725 0.089725
  spline S205 degree 3 poles (24.3328, -487.0306) (24.2243, -486.9421) (23.9997, -486.7589) (23.71, -486.7379) (23.5603, -486.7271) knots 0 0 0 0 0.040971 0.08482 0.08482 0.08482 0.08482
  spline S206 degree 3 poles (23.5603, -486.7271) (23.4646, -486.7322) (23.2773, -486.7423) (23.1078, -486.8225) (23.0248, -486.8618) knots 0 0 0 0 0.028423 0.055689 0.055689 0.055689 0.055689
  spline S207 degree 3 poles (23.0248, -486.8618) (22.9499, -486.9093) (22.8031, -487.0026) (22.7001, -487.1427) (22.6496, -487.2114) knots 0 0 0 0 0.026342 0.051681 0.051681 0.051681 0.051681
  line L381 (22.6496, -487.2114) -> (22.0732, -487.1364)
  line L382 (22.0732, -487.1364) -> (22.5575, -484.5681)
  line L383 (22.5575, -484.5681) -> (25.0438, -484.5681)
  line L384 (25.0438, -484.5681) -> (25.0439, -485.1547)
  line L385 (25.0439, -485.1547) -> (23.0486, -485.1548)
  line L386 (23.0486, -485.1548) -> (22.7792, -486.4986)
  spline S208 degree 3 poles (22.7792, -486.4986) (22.9287, -486.4071) (23.2196, -486.229) (23.559, -486.1992) (23.724, -486.1848) knots 0 0 0 0 0.051785 0.100763 0.100763 0.100763 0.100763
  spline S209 degree 3 poles (23.724, -486.1848) (23.9332, -486.2031) (24.3488, -486.2396) (24.6697, -486.5061) (24.829, -486.6384) knots 0 0 0 0 0.061424 0.122014 0.122014 0.122014 0.122014
  spline S210 degree 3 poles (24.829, -486.6384) (24.9603, -486.8038) (25.2311, -487.1451) (25.2629, -487.5805) (25.2792, -487.8048) knots 0 0 0 0 0.061868 0.127641 0.127641 0.127641 0.127641
  spline S211 degree 3 poles (25.2792, -487.8048) (25.264, -488.0217) (25.2342, -488.4476) (24.999, -488.8035) (24.8836, -488.9781) knots 0 0 0 0 0.064036 0.125703 0.125703 0.125703 0.125703
  spline S212 degree 3 poles (24.8836, -488.9781) (24.7059, -489.1551) (24.3428, -489.5168) (23.8315, -489.5621) (23.5705, -489.5852) knots 0 0 0 0 0.072854 0.148822 0.148822 0.148822 0.148822
  spline S213 degree 3 poles (23.5705, -489.5852) (23.3573, -489.5724) (22.9498, -489.5481) (22.6161, -489.3145) (22.4569, -489.2032) knots 0 0 0 0 0.062678 0.119794 0.119794 0.119794 0.119794
  spline S214 degree 3 poles (22.4569, -489.2032) (22.3283, -489.0628) (22.064, -488.7745) (21.998, -488.3884) (21.9641, -488.1903) knots 0 0 0 0 0.055877 0.114795 0.114795 0.114795 0.114795
  line L387 (28.3829, -488.1731) -> (28.9866, -488.2515)
  spline S215 degree 3 poles (28.9866, -488.2515) (28.9439, -488.4455) (28.8622, -488.8172) (28.6037, -489.0955) (28.4801, -489.2287) knots 0 0 0 0 0.058356 0.111856 0.111856 0.111856 0.111856
  spline S216 degree 3 poles (28.4801, -489.2287) (28.3341, -489.3316) (28.034, -489.5431) (27.6673, -489.5686) (27.4791, -489.5817) knots 0 0 0 0 0.052559 0.107965 0.107965 0.107965 0.107965
  spline S217 degree 3 poles (27.4791, -489.5817) (27.2461, -489.5642) (26.7945, -489.5303) (26.4502, -489.2374) (26.2837, -489.0957) knots 0 0 0 0 0.068154 0.132052 0.132052 0.132052 0.132052
  spline S218 degree 3 poles (26.2837, -489.0957) (26.1521, -488.905) (25.8643, -488.4876) (25.8432, -487.9788) (25.8318, -487.7025) knots 0 0 0 0 0.068157 0.149141 0.149141 0.149141 0.149141
  spline S219 degree 3 poles (25.8318, -487.7025) (25.8381, -487.5172) (25.8501, -487.1647) (25.9695, -486.8332) (26.0261, -486.6759) knots 0 0 0 0 0.055211 0.105055 0.105055 0.105055 0.105055
  spline S220 degree 3 poles (26.0261, -486.6759) (26.0983, -486.539) (26.2405, -486.2693) (26.4934, -486.0995) (26.6179, -486.0159) knots 0 0 0 0 0.04564 0.089884 0.089884 0.089884 0.089884
  spline S221 degree 3 poles (26.6179, -486.0159) (26.7538, -485.9517) (27.0277, -485.8224) (27.3301, -485.8048) (27.4825, -485.7959) knots 0 0 0 0 0.044643 0.089955 0.089955 0.089955 0.089955
  spline S222 degree 3 poles (27.4825, -485.7959) (27.6662, -485.8053) (28.0141, -485.823) (28.3087, -486.0073) (28.4477, -486.0943) knots 0 0 0 0 0.054149 0.102527 0.102527 0.102527 0.102527
  spline S223 degree 3 poles (28.4477, -486.0943) (28.5622, -486.2078) (28.8012, -486.4448) (28.885, -486.7716) (28.9286, -486.9418) knots 0 0 0 0 0.047449 0.099081 0.099081 0.099081 0.099081
  line L388 (28.9286, -486.9418) -> (28.3317, -487.0339)
  spline S224 degree 3 poles (28.3317, -487.0339) (28.3009, -486.9226) (28.2434, -486.7151) (28.0975, -486.5577) (28.0299, -486.4848) knots 0 0 0 0 0.034086 0.063475 0.063475 0.063475 0.063475
  spline S225 degree 3 poles (28.0299, -486.4848) (27.9529, -486.4311) (27.7956, -486.3214) (27.6041, -486.3077) (27.5064, -486.3007) knots 0 0 0 0 0.027619 0.056426 0.056426 0.056426 0.056426
  spline S226 degree 3 poles (27.5064, -486.3007) (27.3597, -486.3137) (27.0706, -486.3394) (26.8576, -486.5362) (26.7526, -486.6332) knots 0 0 0 0 0.04285 0.084486 0.084486 0.084486 0.084486
  spline S227 degree 3 poles (26.7526, -486.6332) (26.6684, -486.7728) (26.4745, -487.0943) (26.467, -487.4718) (26.4627, -487.6854) knots 0 0 0 0 0.048123 0.11083 0.11083 0.11083 0.11083
  spline S228 degree 3 poles (26.4627, -487.6854) (26.4663, -487.9012) (26.4726, -488.2799) (26.6612, -488.6058) (26.7424, -488.7461) knots 0 0 0 0 0.063398 0.111295 0.111295 0.111295 0.111295
  spline S229 degree 3 poles (26.7424, -488.7461) (26.8436, -488.8426) (27.0481, -489.0377) (27.3299, -489.0638) (27.4723, -489.0769) knots 0 0 0 0 0.040675 0.082263 0.082263 0.082263 0.082263
  spline S230 degree 3 poles (27.4723, -489.0769) (27.5867, -489.0687) (27.8095, -489.0527) (27.9888, -488.9199) (28.076, -488.8552) knots 0 0 0 0 0.033628 0.065508 0.065508 0.065508 0.065508
  spline S231 degree 3 poles (28.076, -488.8552) (28.15, -488.7652) (28.3135, -488.5666) (28.3584, -488.3122) (28.3829, -488.1731) knots 0 0 0 0 0.034396 0.07593 0.07593 0.07593 0.07593
  spline S232 degree 3 poles (22.0707, -437.0337) (22.0743, -436.7654) (22.0808, -436.2822) (22.2, -435.8144) (22.2531, -435.6064) knots 0 0 0 0 0.080152 0.144341 0.144341 0.144341 0.144341
  spline S233 degree 3 poles (22.2531, -435.6064) (22.3177, -435.4395) (22.4402, -435.123) (22.6813, -434.885) (22.7953, -434.7724) knots 0 0 0 0 0.052977 0.10048 0.10048 0.10048 0.10048
  spline S234 degree 3 poles (22.7953, -434.7724) (22.9267, -434.6869) (23.2015, -434.508) (23.5295, -434.489) (23.7008, -434.479) knots 0 0 0 0 0.046203 0.096661 0.096661 0.096661 0.096661
  spline S235 degree 3 poles (23.7008, -434.479) (23.8286, -434.4846) (24.0741, -434.4953) (24.2989, -434.5938) (24.4068, -434.641) knots 0 0 0 0 0.037989 0.072993 0.072993 0.072993 0.072993
  spline S236 degree 3 poles (24.4068, -434.641) (24.504, -434.7017) (24.7014, -434.8249) (24.8386, -435.0128) (24.9082, -435.1082) knots 0 0 0 0 0.034048 0.069103 0.069103 0.069103 0.069103
  spline S237 degree 3 poles (24.9082, -435.1082) (24.9715, -435.2192) (25.1055, -435.4541) (25.1796, -435.7144) (25.2186, -435.8517) knots 0 0 0 0 0.038176 0.080832 0.080832 0.080832 0.080832
  spline S238 degree 3 poles (25.2186, -435.8517) (25.2513, -436.0228) (25.3259, -436.4129) (25.3294, -436.8103) (25.3313, -437.0335) knots 0 0 0 0 0.052146 0.118926 0.118926 0.118926 0.118926
  spline S239 degree 3 poles (25.3313, -437.0335) (25.3276, -437.3001) (25.3211, -437.7809) (25.2032, -438.2466) (25.1506, -438.454) knots 0 0 0 0 0.079639 0.143634 0.143634 0.143634 0.143634
  spline S240 degree 3 poles (25.1506, -438.454) (25.0864, -438.621) (24.9646, -438.938) (24.724, -439.1767) (24.6101, -439.2897) knots 0 0 0 0 0.052961 0.100531 0.100531 0.100531 0.100531
  spline S241 degree 3 poles (24.6101, -439.2897) (24.4785, -439.3757) (24.2028, -439.5558) (23.8733, -439.5748) (23.7012, -439.5848) knots 0 0 0 0 0.046338 0.097057 0.097057 0.097057 0.097057
  spline S242 degree 3 poles (23.7012, -439.5848) (23.4749, -439.5655) (23.0337, -439.5278) (22.7188, -439.2176) (22.5654, -439.0664) knots 0 0 0 0 0.065835 0.128409 0.128409 0.128409 0.128409
  spline S243 degree 3 poles (22.5654, -439.0664) (22.4219, -438.7984) (22.0843, -438.1674) (22.0757, -437.4477) (22.0707, -437.0337) knots 0 0 0 0 0.090022 0.211899 0.211899 0.211899 0.211899
  line L389 (28.4896, -438.1724) -> (29.0933, -438.2508)
  spline S244 degree 3 poles (29.0933, -438.2508) (29.0506, -438.4447) (28.9689, -438.8164) (28.7105, -439.0948) (28.5869, -439.228) knots 0 0 0 0 0.058356 0.111856 0.111856 0.111856 0.111856
  spline S245 degree 3 poles (28.5869, -439.228) (28.4408, -439.3309) (28.1407, -439.5424) (27.7741, -439.568) (27.5859, -439.5811) knots 0 0 0 0 0.052559 0.107965 0.107965 0.107965 0.107965
  spline S246 degree 3 poles (27.5859, -439.5811) (27.3528, -439.5636) (26.9012, -439.5297) (26.557, -439.2368) (26.3904, -439.0951) knots 0 0 0 0 0.068154 0.132052 0.132052 0.132052 0.132052
  spline S247 degree 3 poles (26.3904, -439.0951) (26.2589, -438.9044) (25.971, -438.4871) (25.9499, -437.9782) (25.9384, -437.7019) knots 0 0 0 0 0.068157 0.149141 0.149141 0.149141 0.149141
  spline S248 degree 3 poles (25.9384, -437.7019) (25.9447, -437.5167) (25.9567, -437.1642) (26.0761, -436.8326) (26.1327, -436.6753) knots 0 0 0 0 0.055211 0.105055 0.105055 0.105055 0.105055
  spline S249 degree 3 poles (26.1327, -436.6753) (26.2049, -436.5384) (26.3471, -436.2688) (26.6, -436.0989) (26.7244, -436.0153) knots 0 0 0 0 0.04564 0.089884 0.089884 0.089884 0.089884
  spline S250 degree 3 poles (26.7244, -436.0153) (26.8604, -435.9511) (27.1343, -435.8218) (27.4367, -435.8042) (27.589, -435.7953) knots 0 0 0 0 0.044643 0.089955 0.089955 0.089955 0.089955
  spline S251 degree 3 poles (27.589, -435.7953) (27.7727, -435.8046) (28.1206, -435.8224) (28.4152, -436.0067) (28.5542, -436.0936) knots 0 0 0 0 0.054149 0.102527 0.102527 0.102527 0.102527
  spline S252 degree 3 poles (28.5542, -436.0936) (28.6687, -436.2071) (28.9078, -436.4441) (28.9916, -436.7709) (29.0352, -436.9411) knots 0 0 0 0 0.047449 0.099081 0.099081 0.099081 0.099081
  line L390 (29.0352, -436.9411) -> (28.4384, -437.0333)
  spline S253 degree 3 poles (28.4384, -437.0333) (28.4075, -436.9219) (28.35, -436.7144) (28.2041, -436.557) (28.1365, -436.4842) knots 0 0 0 0 0.034086 0.063475 0.063475 0.063475 0.063475
  spline S254 degree 3 poles (28.1365, -436.4842) (28.0595, -436.4305) (27.9022, -436.3207) (27.7107, -436.307) (27.6129, -436.3) knots 0 0 0 0 0.027619 0.056426 0.056426 0.056426 0.056426
  spline S255 degree 3 poles (27.6129, -436.3) (27.4663, -436.3131) (27.1771, -436.3388) (26.9642, -436.5356) (26.8592, -436.6326) knots 0 0 0 0 0.04285 0.084486 0.084486 0.084486 0.084486
  spline S256 degree 3 poles (26.8592, -436.6326) (26.775, -436.7722) (26.5812, -437.0937) (26.5736, -437.4712) (26.5694, -437.6848) knots 0 0 0 0 0.048123 0.11083 0.11083 0.11083 0.11083
  spline S257 degree 3 poles (26.5694, -437.6848) (26.573, -437.9006) (26.5793, -438.2793) (26.7679, -438.6053) (26.8491, -438.7455) knots 0 0 0 0 0.063398 0.111295 0.111295 0.111295 0.111295
  spline S258 degree 3 poles (26.8491, -438.7455) (26.9503, -438.842) (27.1549, -439.0371) (27.4366, -439.0631) (27.579, -439.0763) knots 0 0 0 0 0.040675 0.082263 0.082263 0.082263 0.082263
  spline S259 degree 3 poles (27.579, -439.0763) (27.6934, -439.0681) (27.9163, -439.0521) (28.0955, -438.9192) (28.1827, -438.8546) knots 0 0 0 0 0.033628 0.065508 0.065508 0.065508 0.065508
  spline S260 degree 3 poles (28.1827, -438.8546) (28.2567, -438.7646) (28.4202, -438.5659) (28.4651, -438.3115) (28.4896, -438.1724) knots 0 0 0 0 0.034396 0.07593 0.07593 0.07593 0.07593
  line L391 (22.0661, -388.1903) -> (22.7107, -388.1357)
  spline S261 degree 3 poles (22.7107, -388.1357) (22.7385, -388.2789) (22.7897, -388.5438) (22.9635, -388.7491) (23.0433, -388.8434) knots 0 0 0 0 0.042908 0.079365 0.079365 0.079365 0.079365
  spline S262 degree 3 poles (23.0433, -388.8434) (23.1355, -388.9125) (23.3221, -389.0525) (23.5548, -389.071) (23.6726, -389.0804) knots 0 0 0 0 0.033826 0.068485 0.068485 0.068485 0.068485
  spline S263 degree 3 poles (23.6726, -389.0804) (23.815, -389.0661) (24.1018, -389.0373) (24.3154, -388.8436) (24.4229, -388.7461) knots 0 0 0 0 0.041772 0.0841 0.0841 0.0841 0.0841
  spline S264 degree 3 poles (24.4229, -388.7461) (24.5123, -388.6211) (24.7015, -388.3566) (24.7201, -388.031) (24.7298, -387.8594) knots 0 0 0 0 0.045186 0.095569 0.095569 0.095569 0.095569
  spline S265 degree 3 poles (24.7298, -387.8594) (24.7208, -387.697) (24.7037, -387.3907) (24.5208, -387.1457) (24.4348, -387.0306) knots 0 0 0 0 0.047557 0.089725 0.089725 0.089725 0.089725
  spline S266 degree 3 poles (24.4348, -387.0306) (24.3263, -386.9421) (24.1017, -386.7589) (23.812, -386.7379) (23.6623, -386.7271) knots 0 0 0 0 0.040971 0.08482 0.08482 0.08482 0.08482
  spline S267 degree 3 poles (23.6623, -386.7271) (23.5667, -386.7322) (23.3793, -386.7423) (23.2098, -386.8225) (23.1268, -386.8618) knots 0 0 0 0 0.028423 0.055689 0.055689 0.055689 0.055689
  spline S268 degree 3 poles (23.1268, -386.8618) (23.052, -386.9093) (22.9051, -387.0026) (22.8021, -387.1427) (22.7516, -387.2114) knots 0 0 0 0 0.026342 0.051681 0.051681 0.051681 0.051681
  line L392 (22.7516, -387.2114) -> (22.1752, -387.1364)
  line L393 (22.1752, -387.1364) -> (22.6595, -384.5681)
  line L394 (22.6595, -384.5681) -> (25.1459, -384.5681)
  line L395 (25.1459, -384.5681) -> (25.1459, -385.1547)
  line L396 (25.1459, -385.1547) -> (23.1507, -385.1548)
  line L397 (23.1507, -385.1548) -> (22.8812, -386.4986)
  spline S269 degree 3 poles (22.8812, -386.4986) (23.0307, -386.4071) (23.3216, -386.229) (23.661, -386.1992) (23.826, -386.1848) knots 0 0 0 0 0.051785 0.100763 0.100763 0.100763 0.100763
  spline S270 degree 3 poles (23.826, -386.1848) (24.0352, -386.2031) (24.4508, -386.2396) (24.7717, -386.5061) (24.931, -386.6384) knots 0 0 0 0 0.061424 0.122014 0.122014 0.122014 0.122014
  spline S271 degree 3 poles (24.931, -386.6384) (25.0623, -386.8038) (25.3332, -387.1451) (25.3649, -387.5805) (25.3813, -387.8048) knots 0 0 0 0 0.061868 0.12764 0.12764 0.12764 0.12764
  spline S272 degree 3 poles (25.3813, -387.8048) (25.3661, -388.0217) (25.3362, -388.4476) (25.101, -388.8035) (24.9856, -388.9781) knots 0 0 0 0 0.064036 0.125703 0.125703 0.125703 0.125703
  spline S273 degree 3 poles (24.9856, -388.9781) (24.8079, -389.1551) (24.4449, -389.5168) (23.9336, -389.5621) (23.6726, -389.5852) knots 0 0 0 0 0.072854 0.148822 0.148822 0.148822 0.148822
  spline S274 degree 3 poles (23.6726, -389.5852) (23.4593, -389.5724) (23.0518, -389.5481) (22.7181, -389.3145) (22.559, -389.2032) knots 0 0 0 0 0.062678 0.119794 0.119794 0.119794 0.119794
  spline S275 degree 3 poles (22.559, -389.2032) (22.4303, -389.0628) (22.1661, -388.7745) (22.1, -388.3884) (22.0661, -388.1903) knots 0 0 0 0 0.055877 0.114795 0.114795 0.114795 0.114795
  line L398 (28.485, -388.1731) -> (29.0886, -388.2515)
  spline S276 degree 3 poles (29.0886, -388.2515) (29.046, -388.4455) (28.9642, -388.8172) (28.7058, -389.0955) (28.5822, -389.2287) knots 0 0 0 0 0.058356 0.111856 0.111856 0.111856 0.111856
  spline S277 degree 3 poles (28.5822, -389.2287) (28.4361, -389.3316) (28.136, -389.5431) (27.7693, -389.5686) (27.5812, -389.5817) knots 0 0 0 0 0.052559 0.107965 0.107965 0.107965 0.107965
  spline S278 degree 3 poles (27.5812, -389.5817) (27.3481, -389.5642) (26.8965, -389.5303) (26.5523, -389.2374) (26.3857, -389.0957) knots 0 0 0 0 0.068154 0.132052 0.132052 0.132052 0.132052
  spline S279 degree 3 poles (26.3857, -389.0957) (26.2542, -388.905) (25.9663, -388.4876) (25.9452, -387.9788) (25.9338, -387.7025) knots 0 0 0 0 0.068157 0.149141 0.149141 0.149141 0.149141
  spline S280 degree 3 poles (25.9338, -387.7025) (25.9401, -387.5172) (25.9521, -387.1647) (26.0715, -386.8332) (26.1282, -386.6759) knots 0 0 0 0 0.055211 0.105055 0.105055 0.105055 0.105055
  spline S281 degree 3 poles (26.1282, -386.6759) (26.2004, -386.539) (26.3426, -386.2693) (26.5954, -386.0995) (26.7199, -386.0159) knots 0 0 0 0 0.04564 0.089884 0.089884 0.089884 0.089884
  spline S282 degree 3 poles (26.7199, -386.0159) (26.8558, -385.9517) (27.1297, -385.8224) (27.4322, -385.8048) (27.5845, -385.7959) knots 0 0 0 0 0.044643 0.089955 0.089955 0.089955 0.089955
  spline S283 degree 3 poles (27.5845, -385.7959) (27.7682, -385.8053) (28.1161, -385.823) (28.4107, -386.0073) (28.5497, -386.0943) knots 0 0 0 0 0.054149 0.102527 0.102527 0.102527 0.102527
  spline S284 degree 3 poles (28.5497, -386.0943) (28.6642, -386.2078) (28.9032, -386.4448) (28.987, -386.7716) (29.0306, -386.9418) knots 0 0 0 0 0.047449 0.099081 0.099081 0.099081 0.099081
  line L399 (29.0306, -386.9418) -> (28.4338, -387.0339)
  spline S285 degree 3 poles (28.4338, -387.0339) (28.4029, -386.9226) (28.3454, -386.7151) (28.1995, -386.5577) (28.1319, -386.4848) knots 0 0 0 0 0.034086 0.063475 0.063475 0.063475 0.063475
  spline S286 degree 3 poles (28.1319, -386.4848) (28.0549, -386.4311) (27.8976, -386.3214) (27.7061, -386.3077) (27.6084, -386.3007) knots 0 0 0 0 0.027619 0.056426 0.056426 0.056426 0.056426
  spline S287 degree 3 poles (27.6084, -386.3007) (27.4617, -386.3137) (27.1726, -386.3394) (26.9596, -386.5362) (26.8546, -386.6332) knots 0 0 0 0 0.04285 0.084486 0.084486 0.084486 0.084486
  spline S288 degree 3 poles (26.8546, -386.6332) (26.7705, -386.7728) (26.5766, -387.0943) (26.569, -387.4718) (26.5648, -387.6854) knots 0 0 0 0 0.048123 0.11083 0.11083 0.11083 0.11083
  spline S289 degree 3 poles (26.5648, -387.6854) (26.5683, -387.9012) (26.5746, -388.2799) (26.7633, -388.6058) (26.8444, -388.7461) knots 0 0 0 0 0.063398 0.111295 0.111295 0.111295 0.111295
  spline S290 degree 3 poles (26.8444, -388.7461) (26.9456, -388.8426) (27.1502, -389.0377) (27.4319, -389.0638) (27.5743, -389.0769) knots 0 0 0 0 0.040675 0.082263 0.082263 0.082263 0.082263
  spline S291 degree 3 poles (27.5743, -389.0769) (27.6887, -389.0687) (27.9115, -389.0527) (28.0908, -388.9199) (28.178, -388.8552) knots 0 0 0 0 0.033628 0.065508 0.065508 0.065508 0.065508
  spline S292 degree 3 poles (28.178, -388.8552) (28.2521, -388.7653) (28.4155, -388.5666) (28.4604, -388.3122) (28.485, -388.1731) knots 0 0 0 0 0.034396 0.07593 0.07593 0.07593 0.07593